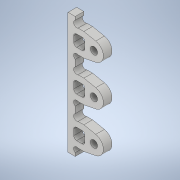
# Autodesk Inventor part: アームユニット底板締結パーツ3t用
Saved by Autodesk Inventor 2020.1 (Build 241239000, 239)
## iProperties
Created: 2018-11-28
Part Number: アームユニット底板締結パーツ3t用
Material: アルミニウム 2014-T4
Document SubType Name: Modeling
Designer: 雪村
Density: 2.8 g/cm^3
Appearance: サテン
Mass: 2.0212 g
Surface Area: 10.9167 cm^2
Volume: 0.721856 cm^3
Description: アルミ2000 3t
Author: 雪村
Autodesk Inventor part; units mm, degrees
ref_plane "YZ Plane" through (0, 0, 0) normal (1, 0, 0) x (0, 1, 0)
ref_plane "XZ Plane" through (0, 0, 0) normal (0, 1, 0) x (-1, 0, 0)
ref_plane "XY Plane" through (0, 0, 0) normal (0, 0, 1) x (1, 0, 0)
sketch "スケッチ1" plane through (0, 0, 0) normal (0, 0, 1) x (1, 0, 0)
  line L0 (-7, -29) -> (-7, -27)
  arc A0 (-6, -26) -> (-7, -27) centre (-6, -27) ccw
  line L1 (-6, -26) -> (-4.1307, -26)
  arc A1 (-3.1588, -27.2353) -> (-4.1307, -26) centre (-4.1307, -27) ccw
  arc A2 (-3.1588, -27.2353) -> (-3.1588, -28.7647) centre (0, -28) ccw
  arc A3 (-4.1307, -30) -> (-3.1588, -28.7647) centre (-4.1307, -29) ccw
  line L2 (-4.1307, -30) -> (-6, -30)
  arc A4 (-7, -29) -> (-6, -30) centre (-6, -29) ccw
  arc A5 (-6.5, -22.1534) -> (-5.5, -24) centre (-6, -23.0767) ccw
  line L3 (-6.5, -21) -> (-6.5, -22.1534)
  line L4 (-9, -21) -> (-6.5, -21)
  line L5 (-9, -35) -> (-9, -21)
  line L6 (-6.5, -35) -> (-9, -35)
  line L7 (-6.5, -33.8466) -> (-6.5, -35)
  arc A6 (-5.5, -32) -> (-6.5, -33.8466) centre (-6, -32.9233) ccw
  line L8 (-3.5, -32) -> (-5.5, -32)
  line L9 (0.6267, -31.189) -> (-3.5, -32)
  arc A7 (0.6267, -31.189) -> (0.6267, -24.811) centre (0, -28) ccw
  line L10 (-3.5, -24) -> (0.6267, -24.811)
  line L11 (-5.5, -24) -> (-3.5, -24)
  circle A8 centre (0, -28) radius 1.25
  line L12 (-7, -15) -> (-7, -13)
  arc A9 (-6, -12) -> (-7, -13) centre (-6, -13) ccw
  line L13 (-6, -12) -> (-4.1307, -12)
  arc A10 (-3.1588, -13.2353) -> (-4.1307, -12) centre (-4.1307, -13) ccw
  arc A11 (-3.1588, -13.2353) -> (-3.1588, -14.7647) centre (0, -14) ccw
  arc A12 (-4.1307, -16) -> (-3.1588, -14.7647) centre (-4.1307, -15) ccw
  line L14 (-4.1307, -16) -> (-6, -16)
  arc A13 (-7, -15) -> (-6, -16) centre (-6, -15) ccw
  arc A14 (-6.5, -8.1534) -> (-5.5, -10) centre (-6, -9.0767) ccw
  line L15 (-6.5, -7) -> (-6.5, -8.1534)
  line L16 (-9, -7) -> (-6.5, -7)
  line L17 (-9, -21) -> (-9, -7)
  line L18 (-6.5, -21) -> (-9, -21)
  line L19 (-6.5, -19.8466) -> (-6.5, -21)
  arc A15 (-5.5, -18) -> (-6.5, -19.8466) centre (-6, -18.9233) ccw
  line L20 (-3.5, -18) -> (-5.5, -18)
  line L21 (0.6267, -17.189) -> (-3.5, -18)
  arc A16 (0.6267, -17.189) -> (0.6267, -10.811) centre (0, -14) ccw
  line L22 (-3.5, -10) -> (0.6267, -10.811)
  line L23 (-5.5, -10) -> (-3.5, -10)
  circle A17 centre (0, -14) radius 1.25
  line L24 (-7, -1) -> (-7, 1)
  arc A18 (-6, 2) -> (-7, 1) centre (-6, 1) ccw
  line L25 (-6, 2) -> (-4.1307, 2)
  arc A19 (-3.1588, 0.7647) -> (-4.1307, 2) centre (-4.1307, 1) ccw
  arc A20 (-3.1588, 0.7647) -> (-3.1588, -0.7647) centre (0, 0) ccw
  arc A21 (-4.1307, -2) -> (-3.1588, -0.7647) centre (-4.1307, -1) ccw
  line L26 (-4.1307, -2) -> (-6, -2)
  arc A22 (-7, -1) -> (-6, -2) centre (-6, -1) ccw
  arc A23 (-6.5, 5.8466) -> (-5.5, 4) centre (-6, 4.9233) ccw
  line L27 (-6.5, 7) -> (-6.5, 5.8466)
  line L28 (-9, 7) -> (-6.5, 7)
  line L29 (-9, -7) -> (-9, 7)
  line L30 (-6.5, -7) -> (-9, -7)
  line L31 (-6.5, -5.8466) -> (-6.5, -7)
  arc A24 (-5.5, -4) -> (-6.5, -5.8466) centre (-6, -4.9233) ccw
  line L32 (-3.5, -4) -> (-5.5, -4)
  line L33 (0.6267, -3.189) -> (-3.5, -4)
  arc A25 (0.6267, -3.189) -> (0.6267, 3.189) centre (0, 0) ccw
  line L34 (-3.5, 4) -> (0.6267, 3.189)
  line L35 (-5.5, 4) -> (-3.5, 4)
  circle A26 centre (0, 0) radius 1.25
  constraints: 72 end point, 48 point on circle, 27 centre point, 17 horizontal, 12 vertical, 117 other
extrude "押し出し1" add sketch "スケッチ1" along normal blind 3
